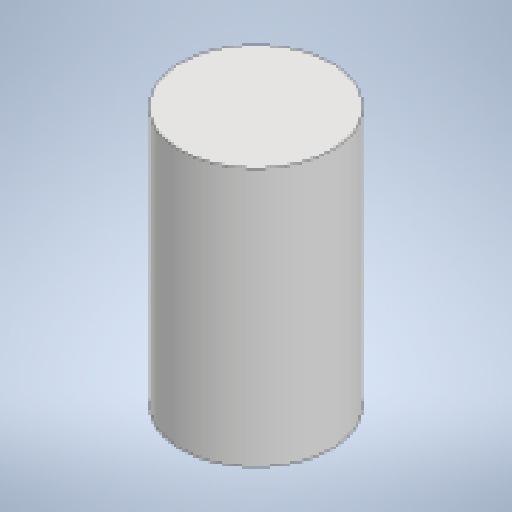
# Autodesk Inventor part: Spindle
Saved by Autodesk Inventor 2023 (Build 270158000, 158)
## iProperties
Created: 2022-05-05
Part Number: Spindle
Material: Generic
Document SubType Name: Modeling
Designer: plebbb
Density: 1 g/cm^3
Appearance: Default
Author: plebbb
Autodesk Inventor part; units mm, degrees
ref_plane "YZ Plane" through (0, 0, 0) normal (1, 0, 0) x (0, 1, 0)
ref_plane "XZ Plane" through (0, 0, 0) normal (0, 1, 0) x (-1, 0, 0)
ref_plane "XY Plane" through (0, 0, 0) normal (0, 0, 1) x (1, 0, 0)
sketch "Sketch1" plane through (0, 0, 0) normal (0, 0, 1) x (1, 0, 0)
  line L0 (0, 0) -> (44.45, 0)
  line L1 (44.45, 0) -> (44.45, 152.4)
  line L2 (44.45, 152.4) -> (0, 152.4)
  line L3 (0, 152.4) -> (0, 0)
  line L4 (4.7625, 0) -> (0, 0)
  line L5 (0, 0) -> (0, -76.2)
  line L6 (0, -76.2) -> (4.7625, -76.2)
  line L7 (4.7625, -76.2) -> (4.7625, 0)
  dimension "d0" = 44.45
  dimension "d1" = 152.4
  dimension "d3" = 4.7625
  dimension "d4" = 76.2
  constraints: 16 end point, 4 parallel, 2 horizontal, 2 perpendicular, 1 point on line
  measures "d0" distance of L1.end L2.end
  measures "d1" distance of L0.end L1.end
  measures "d3" distance of L5.end L6.end
  measures "d4" distance of L6.end L4.start
revolve "Revolution1" add sketch "Sketch1" angle 360 about axis through (0, 152.4, 0) along (0, -1, 0)
body "Solid1"
